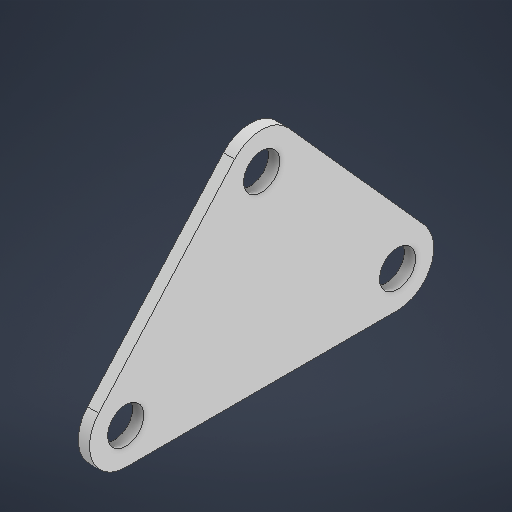
# Autodesk Inventor part: RockerRear
Saved by Autodesk Inventor 2026.2 (Build 302298010, 298A)
## iProperties
Created: 2026-08-01
Part Number: RockerRear
Material: Generic
Document SubType Name: Modeling
Designer: tasle
Density: 1 g/cm^3
Appearance: Default
Author: tasle
Autodesk Inventor part; units mm, degrees
ref_plane "YZ Plane" through (0, 0, 0) normal (1, 0, 0) x (0, 1, 0)
ref_plane "XZ Plane" through (0, 0, 0) normal (0, 1, 0) x (-1, 0, 0)
ref_plane "XY Plane" through (0, 0, 0) normal (0, 0, 1) x (1, 0, 0)
sketch "Sketch1" plane through (0, 0, 0) normal (1, 0, 0) x (0, 1, 0)
  line L0 (0, 30) -> (0, -30)
  line L1 (0, -30) -> (33.541, 0)
  line L2 (33.541, 0) -> (0, 30)
  circle A0 centre (33.541, 0) radius 4
  circle A1 centre (33.541, 0) radius 8
  circle A2 centre (0, -30) radius 4
  circle A3 centre (0, -30) radius 8
  circle A4 centre (0, 30) radius 4
  circle A5 centre (0, 30) radius 8
  line L3 (5.3333, 35.9628) -> (38.8744, 5.9628)
  line L4 (38.8744, -5.9628) -> (5.3333, -35.9628)
  line L5 (-8, -30) -> (-8, 30)
  point P0 (0, 0)
  dimension "d0" = 60
  dimension "d1" = 45
  dimension "d2" = 8
  dimension "d3" = 16
  dimension "d4" = 8
  dimension "d5" = 16
  dimension "d6" = 8
  dimension "d7" = 16
  constraints: 12 end point, 6 centre point, 6 coincident, 6 point on circle, 4 tangent, 2 vertical, 1 horizontal alignment, 1 midpoint, 1 parallel
  measures "d0" distance of L0.start L0.end
  measures "d1" distance of L0.end L1.end
  measures "d2" diameter of A0
  measures "d3" diameter of A1
  measures "d4" diameter of A2
  measures "d5" diameter of A3
  measures "d6" diameter of A4
  measures "d7" diameter of A5
extrude "Extrusion1" add sketch "Sketch1" along normal blind 2.5 contours A4 L2 A5 L0 | L0 A5 L2 A4 | A5 L2 A1 L1 A3 L0 | L0 A3 L5 A5 | A5 L3 A1 L2 | A3 L1 A2 L0 | L0 A2 L1 A3 | A1 L1 A0 L2 | L2 A0 L1 A1 | L1 A1 L4 A3
body "Solid1"
